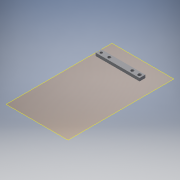
# Autodesk Inventor part: 25_Adapter_FAn
Saved by Autodesk Inventor 2016 (Build 200138000, 138)
## iProperties
Created: 2016-12-10
Part Number: 25_Adapter_FAn
Material: Generisch
Document SubType Name: Modeling
Designer: Bene
Density: 1 g/cm^3
Appearance: Vorgabe
Author: Bene
Autodesk Inventor part; units mm, degrees
ref_plane "YZ Plane" through (0, 0, 0) normal (1, 0, 0) x (0, 1, 0)
ref_plane "XZ Plane" through (0, 0, 0) normal (0, 1, 0) x (-1, 0, 0)
ref_plane "XY Plane" through (0, 0, 0) normal (0, 0, 1) x (1, 0, 0)
ref_plane "Arbeitsebene1" through (0, 0, 0) normal (0, 0, 1) x (1, 0, 0)
sketch "Skizze1" plane through (0, 0, 0) normal (0, 0, 1) x (1, 0, 0)
  circle A0 centre (21.7974, 53.3662) radius 2.25 projected
  circle A1 centre (-31.2026, 53.3662) radius 1.75 projected
  line L0 (25.7974, 2.3662) -> (25.7974, 69.3662) projected
  line L1 (-35.2026, 69.3662) -> (-35.2026, -29.0237) projected
  line L2 (25.7974, 49.3662) -> (-35.2026, 49.3662)
  line L3 (-35.2026, 49.3662) -> (-35.2026, 57.3662)
  line L4 (-35.2026, 57.3662) -> (25.7974, 57.3662)
  line L5 (25.7974, 57.3662) -> (25.7974, 49.3662)
  circle A2 centre (11.7974, 53.3662) radius 2
  circle A3 centre (-20.2026, 53.3662) radius 2
  point P0 (0, 0)
  dimension "d0" = 4
  dimension "d1" = 4
  dimension "d2" = 4
  dimension "d3" = 4
  dimension "d4" = 32
  dimension "d5" = 10
  constraints: 8 end point, 2 centre point, 2 parallel, 2 point on line, 1 horizontal, 1 perpendicular
  measures "d0" distance from line of A0.centre L2
  measures "d1" distance from line of A0.centre L4
  measures "d2" diameter of A2
  measures "d3" diameter of A3
  measures "d4" distance of A3.centre A2.centre
  measures "d5" distance of A2.centre A0.centre
extrude "Extrusion1" add sketch "Skizze1" along normal blind 4
